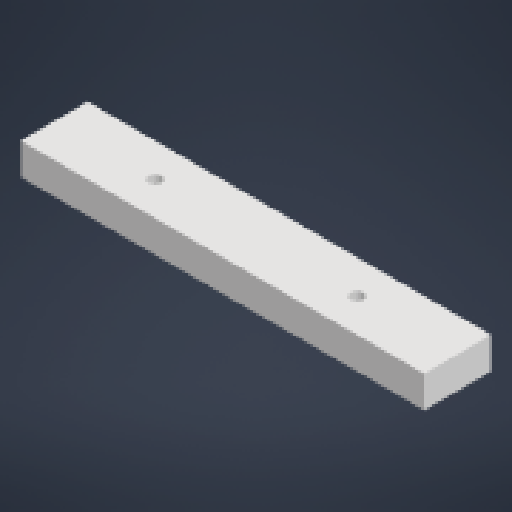
# Autodesk Inventor part: flat
Saved by Autodesk Inventor 2023 (Build 270158000, 158)
## iProperties
Created: 2023-01-24
Part Number: flat
Material: Generic
Document SubType Name: Modeling
Designer: Blank Slate
Density: 1 g/cm^3
Appearance: Default
Author: Blank Slate
Autodesk Inventor part; units mm, degrees
ref_plane "YZ Plane" through (0, 0, 0) normal (1, 0, 0) x (0, 1, 0)
ref_plane "XZ Plane" through (0, 0, 0) normal (0, 1, 0) x (-1, 0, 0)
ref_plane "XY Plane" through (0, 0, 0) normal (0, 0, 1) x (1, 0, 0)
sketch "Sketch1" plane through (0, 0, 0) normal (0, 1, 0) x (-1, 0, 0)
  line L0 (0, 0) -> (-152.4, 0)
  line L1 (-152.4, 0) -> (-152.4, -25.4)
  line L2 (-152.4, -25.4) -> (0, -25.4)
  line L3 (0, -25.4) -> (0, 0)
  line L4 (-152.4, -12.7) -> (0, -12.7) construction
  line L5 (-152.4, -12.7) -> (-114.3, -12.7)
  circle A0 centre (-114.3, -12.7) radius 2.3813
  line L6 (-76.2, 0) -> (-76.2, -25.4) construction
  circle A1 centre (-38.1, -12.7) radius 2.3813
  dimension "d0" = 152.4
  dimension "d1" = 25.4
  dimension "d10" = 38.1
  dimension "d11" = 4.7625
  constraints: 14 end point, 4 midpoint, 2 centre point, 2 coincident, 2 parallel, 2 symmetric about line, 1 horizontal, 1 perpendicular, 1 point on line, 1 other
  measures "d0" distance of L2.end L1.end
  measures "d1" distance of L1.end L0.end
  measures "d10" distance of L4.start L5.end
  measures "d11" diameter of A0
extrude "Extrusion1" add sketch "Sketch1" along normal blind 11.938
body "Solid1"
